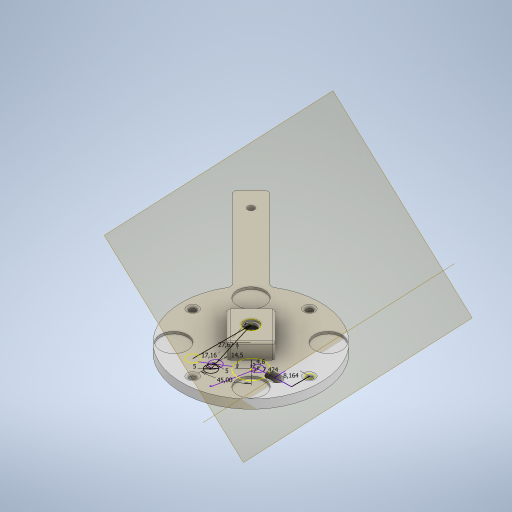
# Autodesk Inventor part: lens_plate
Saved by Autodesk Inventor 2024 (Build 280153000, 153)
## iProperties
Created: 2024-05-03
Part Number: lens_plate
Material: Generic
Document SubType Name: Modeling
Designer: david
Density: 1 g/cm^3
Appearance: Default
Author: david
Autodesk Inventor part; units mm, degrees
ref_plane "YZ Plane" through (0, 0, 0) normal (1, 0, 0) x (0, 1, 0)
ref_plane "XZ Plane" through (0, 0, 0) normal (0, 1, 0) x (-1, 0, 0)
ref_plane "XY Plane" through (0, 0, 0) normal (0, 0, 1) x (1, 0, 0)
sketch "Sketch1" plane through (0, 0, 0) normal (0, 1, 0) x (-1, 0, 0)
  circle A0 centre (0, 0) radius 31.5
  dimension "d0" = 63
  constraints: 1 centre point, 1 coincident
  measures "d0" diameter of A0
extrude "Plate" add sketch "Sketch1" along normal blind 4
sketch "Sketch2" plane through (0, 4, 0) normal (0, 1, 0) x (1, 0, 0)
  circle A0 centre (0, 0) radius 6.65
  dimension "d3" = 13.3
  constraints: 1 centre point, 1 coincident
  measures "d3" diameter of A0
extrude "Lens hole" cut sketch "Sketch2" against normal blind 2
sketch "Sketch3" plane through (0, 2, 0) normal (0, 1, 0) x (1, 0, 0)
  circle A0 centre (0, 0) radius 5
  dimension "d6" = 10
  constraints: 1 centre point, 1 coincident
  measures "d6" diameter of A0
extrude "Optical hole" cut sketch "Sketch3" against normal blind 2
sketch "Sketch4" plane through (0, 4, 0) normal (0, 1, 0) x (1, 0, 0)
  circle A0 centre (0, 0) radius 31.5 projected
  line L0 (0, -31.5) -> (0, -26.5)
  circle A1 centre (0, -26.5) radius 1.55
  circle A2 centre (26.5, 0) radius 1.55
  circle A3 centre (0, 26.5) radius 1.55
  circle A4 centre (-26.5, 0) radius 1.55
  dimension "d9" = 5
  dimension "d10" = 3.1
  dimension "d13" = 360
  constraints: 4 centre point, 2 end point, 1 coincident, 1 vertical, 1 vertical alignment, 10 other
  measures "d9" distance of L0.start L0.end
  measures "d10" diameter of A1
extrude "Screw holes" cut sketch "Sketch4" against normal blind 4 contours A1 | A2 | A3 | A4
sketch "Sketch6" plane through (0, 0, 0) normal (1, 0, 0) x (0, 1, 0)
  point P0 (0, 0)
sketch "Sketch7" plane through (0, 4, 0) normal (0, 1, 0) x (1, 0, 0)
  circle A0 centre (0, 0) radius 5 projected
  circle A1 centre (0, 0) radius 6.65 projected
  line L0 (0, 0) -> (0, 6.65)
  line L1 (0, 0) -> (-5.4801, 5.4801)
  line L2 (-5.4801, 5.4801) -> (0, 10.9602)
  line L3 (0, 10.9602) -> (-1.4142, 12.3744)
  line L4 (-1.4142, 12.3744) -> (-12.3744, 1.4142)
  line L5 (-12.3744, 1.4142) -> (-10.9602, 0)
  line L6 (-10.9602, 0) -> (-5.4801, 5.4801)
  line L7 (0, 0) -> (5.4801, -5.4801)
  line L8 (5.4801, -5.4801) -> (10.9602, 0)
  line L9 (10.9602, 0) -> (12.3744, -1.4142)
  line L10 (12.3744, -1.4142) -> (1.4142, -12.3744)
  line L11 (1.4142, -12.3744) -> (0, -10.9602)
  line L12 (5.4801, -5.4801) -> (0, -10.9602)
  dimension "d25" = 7.75
  dimension "d26" = 45
  dimension "d27" = 2
  dimension "d28" = 15.5
  dimension "d29" = 7.75
  dimension "d30" = 2
  dimension "d31" = 15.5
  constraints: 26 end point, 7 perpendicular, 3 point on line, 1 vertical, 1 vertical alignment, 1 other
  measures "d25" distance of L0.start L1.end
  measures "d26" angle of L1 L0
  measures "d27" distance of L2.end L3.end
  measures "d28" distance of L3.end L4.end
  measures "d29" distance of L0.start L7.end
  measures "d30" distance of L8.end L9.end
  measures "d31" distance of L9.end L10.end
extrude "Extrusion6" add sketch "Sketch7" along normal blind 5 contours L6 L5 L4 L3 L2 | L8 L9 L10 L11 L12
sketch "Sketch8" plane through (0, 9, 0) normal (0, 1, 0) x (1, 0, 0)
  line L0 (0, 10.9602) -> (-1.4142, 12.3744) projected
  line L1 (-10.9602, 0) -> (-12.3744, 1.4142) projected
  line L2 (-1.4142, 12.3744) -> (-12.3744, 1.4142)
  line L3 (1.4142, -12.3744) -> (12.3744, -1.4142) projected
  line L4 (-12.3744, 1.4142) -> (1.4142, -12.3744)
  line L5 (1.4142, -12.3744) -> (12.3744, -1.4142)
  line L6 (12.3744, -1.4142) -> (-1.4142, 12.3744)
  point P0 (0, 0)
  constraints: 8 end point, 3 perpendicular, 1 collinear
extrude "Extrusion7" add sketch "Sketch8" along normal blind 2
sketch "Sketch9" plane through (0, 11, 0) normal (0, 1, 0) x (1, 0, 0)
  circle A0 centre (0, 0) radius 3.3
  dimension "d36" = 6.6
  constraints: 1 centre point, 1 coincident
  measures "d36" diameter of A0
extrude "Extrusion8" cut sketch "Sketch9" against normal blind 1
sketch "Sketch10" plane through (0, 10, 0) normal (0, 1, 0) x (1, 0, 0)
  circle A0 centre (0, 0) radius 2.5
  dimension "d39" = 5
  constraints: 1 centre point, 1 coincident
  measures "d39" diameter of A0
extrude "Extrusion9" cut sketch "Sketch10" against normal blind 1
fillet "Fillet1" radius 1 18 edges at (-6.8943, 11, -6.8943) (6.8943, 11, 6.8943) (-5.4801, 11, 5.4801) (5.4801, 11, -5.4801) (1.4142, 7.5, 12.3744) (-12.3744, 7.5, -1.4142) (-1.4142, 7.5, -12.3744) (12.3744, 7.5, 1.4142) (10.9602, 6.5, 0) (0, 6.5, -10.9602) (5.4801, 9, -5.4801) (-5.4801, 9, 5.4801) (0, 6.5, 10.9602) (-10.9602, 6.5, 0) (-1.55, 4, -26.5) (24.95, 4, 0) (-1.55, 4, 26.5) (-28.05, 4, 0)
sketch "Sketch11" plane through (0, 4, 0) normal (0, 1, 0) x (1, 0, 0)
  line L0 (0, 0) -> (19.0114, 0)
  circle A0 centre (0, 0) radius 2.5 projected
  line L1 (0, 0) -> (22.2739, 22.2739)
  circle A1 centre (0, 0) radius 31.5 projected
  line L2 (22.2739, 22.2739) -> (17.5362, 17.5362)
  circle A2 centre (17.5362, 17.5362) radius 6.2
  circle A3 centre (-17.5362, 17.5362) radius 6.2
  circle A4 centre (-17.5362, -17.5362) radius 6.2
  circle A5 centre (17.5362, -17.5362) radius 6.2
  dimension "d43" = 45
  dimension "d44" = 6.7
  dimension "d45" = 12.4
  dimension "d48" = 360
  constraints: 6 end point, 4 centre point, 1 coincident, 1 horizontal, 1 point on line, 11 other
  measures "d43" angle of L0 L1
  measures "d44" distance of L1.end L2.end
  measures "d45" diameter of A2
extrude "Magnet holdes" cut sketch "Sketch11" against normal blind 1 contours A2 L1 | L1 A2 | A3 | A4 | A5
sketch "Sketch12" plane through (0, 11, 0) normal (0, 1, 0) x (1, 0, 0)
  circle A0 centre (17.5362, -17.5362) radius 6.2 projected
  line L0 (12.143, -20.5944) -> (2.55, -26.5)
  circle A1 centre (0, -26.5) radius 2.55 projected
  circle A2 centre (7.3465, -23.5472) radius 2.5
  circle A3 centre (0, 0) radius 3.3 projected
  line L1 (0, -26.5) -> (0, 0)
  line L2 (0, 0) -> (8.1638, -26.4383)
  line L3 (0, 0) -> (0, -20.3051)
  circle A4 centre (8.1638, -26.4383) radius 2.5
  dimension "d52" = 5
  dimension "d67" = 27.67
  dimension "d68" = 17.16
  dimension "d69" = 5
  constraints: 8 end point, 2 centre point, 1 coincident, 1 horizontal alignment, 1 midpoint, 1 point on line, 1 vertical, 3 other
  measures "d52" diameter of A2
  measures "d67" distance of L1.end L2.end
  measures "d68" angle of L1 L2
  measures "d69" diameter of A4
sketch "Sketch13" plane through (0, 4, 0) normal (0, 1, 0) x (1, 0, 0)
  point P0 (0, 0)
sketch "Sketch14" plane through (0, 4, 0) normal (0, 1, 0) x (1, 0, 0)
  circle A0 centre (-17.5362, 17.5362) radius 6.2 projected
  circle A1 centre (0, 0) radius 3.3 projected
  line L0 (-17.5362, 17.5362) -> (0, 0)
  line L1 (-17.5362, 17.5362) -> (-13.2936, 21.7789)
  line L2 (-17.5362, 17.5362) -> (-21.7789, 13.2936)
  line L3 (-13.2936, 21.7789) -> (-55.72, 64.2053)
  line L4 (-21.7789, 13.2936) -> (-64.2053, 55.72)
  line L5 (-64.2053, 55.72) -> (-55.72, 64.2053)
  point P0 (-22.8834, 14.3981)
  point P1 (-14.3981, 22.8834)
  dimension "d55" = 6
  dimension "d56" = 6
  dimension "d57" = 60
  constraints: 12 end point, 1 perpendicular
  measures "d55" distance of L0.start L1.end
  measures "d56" distance of L0.start L2.end
  measures "d57" distance of L1.end L3.end
extrude "Extrusion12" add sketch "Sketch14" against normal blind 4 contours A0 L4 L5 L3
sketch "Sketch15" plane through (0, 4, 0) normal (0, 1, 0) x (1, 0, 0)
  line L0 (-64.2053, 55.72) -> (-55.72, 64.2053) projected
  line L1 (-59.9627, 59.9627) -> (-52.8916, 52.8916)
  circle A0 centre (-52.8916, 52.8916) radius 1.5
  point P0 (0, 0)
  dimension "d61" = 10
  dimension "d62" = 3
  constraints: 2 end point, 1 centre point, 1 coincident, 1 midpoint
  measures "d61" distance of L1.start L1.end
  measures "d62" diameter of A0
extrude "Extrusion13" cut sketch "Sketch15" against normal blind 4
fillet "Fillet2" radius 2 4 edges at (-55.72, 2, -64.2053) (-64.2053, 2, -55.72) (-17.6234, 2, -26.1087) (-26.1087, 2, -17.6234)
sketch "Sketch16" plane through (0, 4, 0) normal (0, 1, 0) x (1, 0, 0)
  circle A0 centre (0, 0) radius 5 projected
  line L0 (0, 0) -> (10.253, -10.253)
  line L1 (0, 0) -> (0, -12.3744)
  line L2 (10.253, -10.253) -> (11.6673, -8.8388)
  line L3 (11.6673, -8.8388) -> (8.1638, -26.4383)
  circle A1 centre (11.6673, -8.8388) radius 2.3
  circle A2 centre (26.5, 0) radius 1.55 projected
  line L4 (26.5, 0) -> (26.5, -8.164)
  line L5 (11.6673, -8.8388) -> (26.5, -8.164)
  line L6 (11.6673, -8.8388) -> (19.0836, -8.5014)
  line L7 (19.0836, -8.5014) -> (18.8479, -3.3206)
  dimension "d72" = 14.5
  dimension "d73" = 45
  dimension "d74" = 2
  dimension "d75" = 4.6
  dimension "d76" = 8.164
  dimension "d77" = 7.424
  constraints: 16 end point, 2 vertical, 1 centre point, 1 coincident, 1 perpendicular, 1 point on line
  measures "d72" distance of L0.start L0.end
  measures "d73" angle of L1 L0
  measures "d74" distance of L0.end L2.end
  measures "d75" diameter of A1
  measures "d76" distance of L4.start L4.end
  measures "d77" distance of L5.start L6.end
sketch "Sketch17" plane through (0, 4, 0) normal (0, 1, 0) x (1, 0, 0)
  point P0 (0, 0)
sketch "Sketch18" plane through (0, 0, 0) normal (0, 1, 0) x (-1, 0, 0)
  point P0 (0, 0)
sketch "Sketch19" plane through (0, 0, 0) normal (0, 0, 1) x (1, 0, 0)
  point P0 (0, 0)
ref_plane "Work Plane1" through (19.0836, 4, 8.5014) normal (0.7063761, 0.7071068, -0.0321375) x (-0.0454493, 0, -0.9989666)
sketch "Sketch20" plane through (19.0836, 4, 8.5014) normal (0.7063761, 0.7071068, -0.0321375) x (-0.0454493, 0, -0.9989666)
  circle A0 centre (0, 0) radius 2.5
  point P0 (9.36, 10.3786)
  dimension "d79" = 5
  constraints: 1 centre point
  measures "d79" diameter of A0
extrude "Extrusion15" cut sketch "Sketch20" along normal mid plane 17
body "Solid1"
